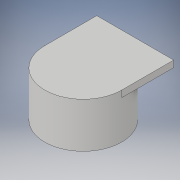
# Autodesk Inventor part: hubholder
Saved by Autodesk Inventor 2019 (Build 230136000, 136)
## iProperties
Created: 2019-08-11
Part Number: hubholder
Material: Generic
Document SubType Name: Modeling
Designer: rob
Density: 1 g/cm^3
Appearance: Default
Author: rob
Autodesk Inventor part; units mm, degrees
ref_plane "YZ Plane" through (0, 0, 0) normal (1, 0, 0) x (0, 1, 0)
ref_plane "XZ Plane" through (0, 0, 0) normal (0, 1, 0) x (-1, 0, 0)
ref_plane "XY Plane" through (0, 0, 0) normal (0, 0, 1) x (1, 0, 0)
sketch "Sketch1" plane through (0, 0, 0) normal (0, 1, 0) x (-1, 0, 0)
  circle A0 centre (0, 0) radius 11.25
  circle A1 centre (0, 0) radius 17.5
  dimension "d0" = 22.5
  dimension "d1" = 35
  constraints: 2 centre point, 2 coincident
  measures "d0" diameter of A0
  measures "d1" diameter of A1
extrude "Extrusion1" add sketch "Sketch1" along normal blind 8
sketch "Sketch2" plane through (0, 8, 0) normal (0, 1, 0) x (1, 0, 0)
  circle A0 centre (0, 0) radius 17.5
  circle A1 centre (0, 0) radius 8.9803
  constraints: 2 centre point, 2 coincident
extrude "Extrusion2" add sketch "Sketch2" along normal blind 9.525
sketch "Sketch3" plane through (0, 17.525, 0) normal (0, 1, 0) x (1, 0, 0)
  circle A0 centre (0, 0) radius 17.5 projected
  line L0 (-17.5, 0) -> (-17.5, 23.6629)
  line L1 (-17.5, 23.6629) -> (17.5, 23.6629)
  line L2 (17.5, 23.6629) -> (17.5, 0)
  arc A1 (-17.5, 0) -> (17.5, 0) centre (0, 0) ccw
  constraints: 6 end point, 2 point on circle, 1 centre point, 1 coincident, 1 horizontal alignment, 1 parallel, 2 other
extrude "Extrusion3" add sketch "Sketch3" along normal blind 3
body "Solid1"
